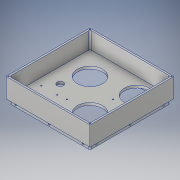
# Autodesk Inventor part: Housing_top
Saved by Autodesk Inventor 2018 (Build 220112000, 112)
## iProperties
Created: 2021-04-22
Part Number: Housing_top
Material: Aluminum 6061
Document SubType Name: Modeling
Designer: Ramana Bharathi
Mass: 926.269 g
Surface Area: 1493.87 cm^2
Volume: 343.063 cm^3
Density: 2.7 g/cm^3
Appearance: Aluminum - Flat
Author: Ramana Bharathi
Autodesk Inventor part; units mm, degrees
ref_plane "YZ Plane" through (0, 0, 0) normal (1, 0, 0) x (0, 1, 0)
ref_plane "XZ Plane" through (0, 0, 0) normal (0, 1, 0) x (-1, 0, 0)
ref_plane "XY Plane" through (0, 0, 0) normal (0, 0, 1) x (1, 0, 0)
sketch "Sketch1" plane through (0, 0, 0) normal (0, 1, 0) x (-1, 0, 0)
  line L0 (0, 0) -> (200, 0)
  line L1 (200, 0) -> (200, -200)
  line L2 (200, -200) -> (0, -200)
  line L3 (0, -200) -> (0, 0)
  dimension "d0" = 200
  dimension "d1" = 200
  constraints: 8 end point, 2 parallel, 1 horizontal, 1 perpendicular
  measures "d0" distance of L1.end L2.end
  measures "d1" distance of L0.end L1.end
extrude "Extrusion1" add sketch "Sketch1" along normal blind 56
sketch "Sketch2" plane through (0, 56, 0) normal (0, 1, 0) x (1, 0, 0)
  line L0 (-4, 4) -> (-196, 4)
  line L1 (-196, 4) -> (-196, 196)
  line L2 (-196, 196) -> (-4, 196)
  line L3 (-4, 196) -> (-4, 4)
  line L4 (0, 0) -> (0, 200) projected
  line L5 (-200, 0) -> (0, 0) projected
  dimension "d4" = 192
  dimension "d5" = 192
  dimension "d6" = 4
  dimension "d7" = 4
  constraints: 8 end point, 2 parallel, 1 horizontal, 1 perpendicular
  measures "d4" distance of L1.end L2.end
  measures "d5" distance of L0.end L1.end
  measures "d6" distance between parallel lines of L4 L3
  measures "d7" distance between parallel lines of L5 L0
extrude "Extrusion2" cut sketch "Sketch2" against normal blind 40
sketch "Sketch3" plane through (0, 0, 0) normal (0, -1, 0) x (1, 0, 0)
  line L0 (-196, -4) -> (-4, -4)
  line L1 (-4, -4) -> (-4, -196)
  line L2 (-4, -196) -> (-196, -196)
  line L3 (-196, -196) -> (-196, -4)
  line L4 (-200, 0) -> (-200, -200) projected
  line L5 (0, 0) -> (-200, 0) projected
  line L6 (0, 0) -> (-200, 0) projected
  line L7 (-200, 0) -> (-200, -200) projected
  line L8 (-200, -200) -> (0, -200) projected
  line L9 (0, -200) -> (0, 0) projected
  line L10 (-8, -8) -> (-192, -8)
  line L11 (-192, -8) -> (-192, -192)
  line L12 (-192, -192) -> (-8, -192)
  line L13 (-8, -192) -> (-8, -8)
  dimension "d10" = 192
  dimension "d11" = 192
  dimension "d12" = 4
  dimension "d13" = 4
  dimension "d16" = 4
  constraints: 16 end point, 4 parallel, 2 perpendicular, 1 horizontal, 3 other
  measures "d10" distance of L1.end L2.end
  measures "d11" distance of L0.end L1.end
  measures "d12" distance between parallel lines of L4 L3
  measures "d13" distance between parallel lines of L0 L5
  measures "d16" distance between parallel lines of L0 L10
extrude "Extrusion3" cut sketch "Sketch3" against normal blind 10
fillet "Fillet1" radius 4 12 edges at (-196, 36, -196) (-196, 36, -4) (-4, 36, -196) (-4, 36, -4) (-4, 5, -4) (-4, 5, -196) (-196, 5, -196) (-196, 5, -4) (-8, 5, -192) (-8, 5, -8) (-192, 5, -192) (-192, 5, -8)
sketch "Sketch8" plane through (0, 16, 0) normal (0, 1, 0) x (1, 0, 0)
  circle A0 centre (-65, 65) radius 40
  line L0 (0, 0) -> (0, 200)
  line L1 (-200, 0) -> (0, 0)
  circle A1 centre (-140, 140) radius 37.5
  line L2 (0, 200) -> (-200, 200)
  line L3 (-200, 200) -> (-200, 0)
  circle A2 centre (-140, 140) radius 55
  line L4 (-185, 78) -> (-135, 78)
  line L5 (-135, 78) -> (-135, 10)
  line L6 (-135, 10) -> (-185, 10)
  line L7 (-185, 10) -> (-185, 78)
  circle A3 centre (-65, 65) radius 50
  circle A4 centre (-65, 65) radius 60
  line L8 (-185, 19) -> (-135, 19)
  line L9 (-135, 19) -> (-135, 69)
  line L10 (-135, 69) -> (-185, 69)
  line L11 (-185, 69) -> (-185, 19)
  circle A5 centre (-140, 140) radius 30
  circle A6 centre (-45, 157) radius 30
  circle A7 centre (-65, 65) radius 30
  circle A8 centre (-160, 89) radius 7.5
  line L12 (0, 0) -> (0, 200) projected
  line L13 (-200, 0) -> (0, 0) projected
  dimension "d152" = 80
  dimension "d153" = 65
  dimension "d154" = 65
  dimension "d155" = 75
  dimension "d156" = 140
  dimension "d157" = 140
  dimension "d158" = 110
  dimension "d159" = 50
  dimension "d160" = 68
  dimension "d161" = 10
  dimension "d162" = 100
  dimension "d163" = 120
  dimension "d164" = 135
  dimension "d165" = 50
  dimension "d166" = 50
  dimension "d167" = 9
  dimension "d168" = 60
  dimension "d169" = 60
  dimension "d170" = 60
  dimension "d171" = 15
  dimension "d172" = 20
  dimension "d173" = 25
  dimension "d174" = 45
  dimension "d175" = 157
  constraints: 24 end point, 9 centre point, 5 coincident, 4 parallel, 3 horizontal, 2 perpendicular, 1 point on line, 1 vertical
  measures "d152" diameter of A0
  measures "d153" distance from line of L0 A0.centre
  measures "d154" distance from line of L1 A0.centre
  measures "d155" diameter of A1
  measures "d156" distance from line of L1 A1.centre
  measures "d157" distance from line of L0 A1.centre
  measures "d158" diameter of A2
  measures "d159" distance of L5.end L6.end
  measures "d160" distance of L4.end L5.end
  measures "d161" distance between parallel lines of L1 L6
  measures "d162" diameter of A3
  measures "d163" diameter of A4
  measures "d164" distance between parallel lines of L0 L5
  measures "d165" distance of L10.end L9.end
  measures "d166" distance of L9.end L8.end
  measures "d167" distance between parallel lines of L8 L6
  measures "d168" diameter of A5
  measures "d169" diameter of A6
  measures "d170" diameter of A7
  measures "d171" diameter of A8
  measures "d172" distance from line of L10 A8.centre
  measures "d173" distance from line of L11 A8.centre
  measures "d174" distance from line of L0 A6.centre
  measures "d175" distance from line of L13 A6.centre
extrude "Extrusion4" cut sketch "Sketch8" against normal through all contours A8 A2 | A2 A8 | A5 | A6 | A7
sketch "Sketch4" plane through (0, 56, 0) normal (0, 1, 0) x (1, 0, 0)
  circle A0 centre (-197, 197) radius 1.5
  line L0 (0, 200) -> (-200, 200) projected
  line L1 (-200, 200) -> (-200, 0) projected
  circle A1 centre (-197, 3) radius 1.5
  line L2 (-200, 0) -> (0, 0) projected
  circle A2 centre (-3, 197) radius 1.5
  line L3 (0, 0) -> (0, 200) projected
  circle A3 centre (-3, 3) radius 1.5
  dimension "d18" = 3
  dimension "d19" = 3
  dimension "d20" = 3
  dimension "d21" = 3
  dimension "d22" = 3
  dimension "d23" = 3
  dimension "d24" = 3
  dimension "d25" = 3
  dimension "d26" = 3
  dimension "d27" = 3
  dimension "d28" = 3
  dimension "d29" = 3
  constraints: 4 centre point
  measures "d18" diameter of A0
  measures "d19" distance from line of L0 A0.centre
  measures "d20" distance from line of L1 A0.centre
  measures "d21" diameter of A1
  measures "d22" distance from line of L1 A1.centre
  measures "d23" distance from line of L2 A1.centre
  measures "d24" diameter of A2
  measures "d25" distance from line of L0 A2.centre
  measures "d26" distance from line of L3 A2.centre
  measures "d27" diameter of A3
  measures "d28" distance from line of L3 A3.centre
  measures "d29" distance from line of L2 A3.centre
hole "Hole1" at (-197, 56, -3) at (-197, 56, -197) at (-3, 56, -197) at (-3, 56, -3) direction (0, -1, 0) diameter 3 depth 5 tip angle 118
sketch "Sketch5" plane through (-4, 0, -8) normal (1, 0, 0) x (0, 0, -1)
  circle A0 centre (11, 5) radius 2
  line L0 (184, 0) -> (0, 0) projected
  circle A1 centre (91, 5) radius 2
  circle A2 centre (171, 5) radius 2
  line L1 (-4, 10) -> (-4, 0) projected
  line L2 (-4, 0) -> (-4, 10) projected
  line L3 (-4, 10) -> (-4, 0) projected
  line L4 (0, 0) -> (0, 10) projected
  dimension "d37" = 4
  dimension "d38" = 5
  dimension "d42" = 80
  dimension "d54" = 11
  constraints: 3 centre point, 1 horizontal, 4 other
  measures "d37" diameter of A0
  measures "d38" distance from line of L0 A0.centre
  measures "d42" distance of A0.centre A1.centre
  measures "d54" distance from line of L4 A0.centre
hole "Hole2" at (-4, 5, -19) at (-4, 5, -99) at (-4, 5, -179) direction (-1, 0, 0) diameter 4 end through all
sketch "Sketch6" plane through (-192, 0, -4) normal (0, 0, 1) x (1, 0, 0)
  circle A0 centre (11, 5) radius 2
  line L0 (182, 0) -> (0, 0)
  line L1 (-4, 0) -> (-4, 10)
  circle A1 centre (91, 5) radius 2
  circle A2 centre (171, 5) radius 2
  line L2 (-4, 10) -> (-4, 0)
  line L3 (-4, 0) -> (-4, 10)
  line L4 (-4, 10) -> (-4, 0)
  line L5 (0, 0) -> (0, 10)
  point P0 (192, 0)
  point P1 (186, 0)
  dimension "d59" = 4
  dimension "d60" = 5
  dimension "d61" = 80
  dimension "d62" = 11
  constraints: 12 end point, 3 centre point, 1 horizontal, 4 other
  measures "d59" diameter of A0
  measures "d60" distance from line of L0 A0.centre
  measures "d61" distance of A0.centre A1.centre
  measures "d62" distance from line of L5 A0.centre
hole "Hole3" at (-181, 5, -4) at (-101, 5, -4) at (-21, 5, -4) direction (0, 0, -1) diameter 4 end through all
sketch "Sketch7" plane through (0, 16, 0) normal (0, 1, 0) x (1, 0, 0)
  line L0 (-200, 200) -> (-200, 0) projected
  line L1 (-200, 0) -> (0, 0) projected
  line L2 (-185, 78) -> (-135, 78)
  line L3 (-135, 78) -> (-135, 10)
  line L4 (-135, 10) -> (-185, 10)
  line L5 (-185, 10) -> (-185, 78)
  line L6 (0, 0) -> (0, 200) projected
  line L7 (-185, 78) -> (-173, 78)
  line L8 (-173, 78) -> (-173, 10)
  line L9 (-173, 10) -> (-185, 10)
  line L10 (-185, 10) -> (-185, 78)
  line L11 (-135, 78) -> (-147, 78)
  line L12 (-147, 78) -> (-147, 10)
  line L13 (-147, 10) -> (-135, 10)
  line L14 (-135, 10) -> (-135, 78)
  circle A0 centre (-179, 63) radius 2
  circle A1 centre (-179, 25) radius 2
  circle A2 centre (-141, 63) radius 2
  circle A3 centre (-141, 25) radius 2
  circle A4 centre (-65, 65) radius 60
  circle A5 centre (-65, 65) radius 55
  circle A6 centre (-65, 120) radius 2
  circle A7 centre (-120, 65) radius 2
  circle A8 centre (-65, 10) radius 2
  circle A9 centre (-10, 65) radius 2
  dimension "d106" = 110
  dimension "d74" = 50
  dimension "d75" = 68
  dimension "d76" = 10
  dimension "d79" = 135
  dimension "d80" = 12
  dimension "d81" = 68
  dimension "d82" = 12
  dimension "d83" = 68
  dimension "d84" = 4
  dimension "d85" = 4
  dimension "d86" = 4
  dimension "d87" = 4
  dimension "d88" = 15
  dimension "d89" = 15
  dimension "d90" = 15
  dimension "d91" = 15
  dimension "d92" = 6
  dimension "d93" = 6
  dimension "d94" = 6
  dimension "d95" = 6
  dimension "d103" = 120
  dimension "d104" = 65
  dimension "d105" = 65
  dimension "d107" = 4
  dimension "d110" = 360
  constraints: 24 end point, 9 centre point, 6 parallel, 3 horizontal, 3 perpendicular, 1 coincident, 1 vertical alignment, 11 other
  measures "d74" distance of L3.end L4.end
  measures "d75" distance of L2.end L3.end
  measures "d76" distance between parallel lines of L1 L4
  measures "d79" distance between parallel lines of L6 L3
  measures "d80" distance of L8.end L9.end
  measures "d81" distance of L7.end L8.end
  measures "d82" distance of L13.end L12.end
  measures "d83" distance of L12.end L11.end
  measures "d84" diameter of A0
  measures "d85" diameter of A1
  measures "d86" diameter of A2
  measures "d87" diameter of A3
  measures "d88" distance from line of L7 A0.centre
  measures "d89" distance from line of L2 A2.centre
  measures "d90" distance from line of L9 A1.centre
  measures "d91" distance from line of L13 A3.centre
  measures "d92" distance from line of L5 A0.centre
  measures "d93" distance from line of L10 A1.centre
  measures "d94" distance from line of L3 A2.centre
  measures "d95" distance from line of L14 A3.centre
  measures "d103" diameter of A4
  measures "d104" distance from line of L1 A4.centre
  measures "d105" distance from line of L6 A4.centre
  measures "d107" diameter of A6
hole "Hole4" at (-179, 16, -63) at (-141, 16, -63) at (-179, 16, -25) at (-141, 16, -25) at (-65, 16, -120) at (-120, 16, -65) at (-65, 16, -10) at (-10, 16, -65) direction (0, -1, 0) diameter 3 depth 5 tip angle 118
thread "Thread1" size "M3x0.5" class "6H" standard "ANSI Metric M Profile" full length
thread "Thread2" size "M3x0.5" class "6H" standard "ANSI Metric M Profile" full length
thread "Thread3" size "M3x0.5" class "6H" standard "ANSI Metric M Profile" full length
thread "Thread4" size "M3x0.5" class "6H" standard "ANSI Metric M Profile" full length
thread "Thread5" size "M3x0.5" class "6H" standard "ANSI Metric M Profile" full length
thread "Thread6" size "M3x0.5" class "6H" standard "ANSI Metric M Profile" full length
thread "Thread7" size "M3x0.5" class "6H" standard "ANSI Metric M Profile" full length
thread "Thread8" size "M3x0.5" class "6H" standard "ANSI Metric M Profile" full length
thread "Thread9" size "M4x0.7" class "6H" standard "ANSI Metric M Profile" full length
thread "Thread10" size "M4x0.7" class "6H" standard "ANSI Metric M Profile" full length
thread "Thread11" size "M4x0.7" class "6H" standard "ANSI Metric M Profile" full length
thread "Thread12" size "M4x0.7" class "6H" standard "ANSI Metric M Profile" full length
thread "Thread13" size "M4x0.7" class "6H" standard "ANSI Metric M Profile" full length
thread "Thread14" size "M4x0.7" class "6H" standard "ANSI Metric M Profile" full length
thread "Thread15" size "M4x0.7" class "6H" standard "ANSI Metric M Profile" full length
thread "Thread16" size "M4x0.7" class "6H" standard "ANSI Metric M Profile" full length
thread "Thread17" size "M4x0.7" class "6H" standard "ANSI Metric M Profile" full length
thread "Thread18" size "M4x0.7" class "6H" standard "ANSI Metric M Profile" full length
thread "Thread19" size "M4x0.7" class "6H" standard "ANSI Metric M Profile" full length
thread "Thread20" size "M4x0.7" class "6H" standard "ANSI Metric M Profile" full length
thread "Thread21" size "M3x0.5" class "6H" standard "ANSI Metric M Profile" full length
thread "Thread22" size "M3x0.5" class "6H" standard "ANSI Metric M Profile" full length
thread "Thread23" size "M3x0.5" class "6H" standard "ANSI Metric M Profile" full length
thread "Thread24" size "M3x0.5" class "6H" standard "ANSI Metric M Profile" full length
body "Solid1"
